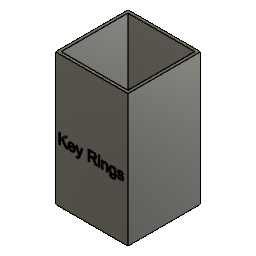
10-32 Box v2 (Autodesk Fusion 360 design; units mm, degrees)
Autodesk Fusion 360 part; units mm, degrees
sketch "Sketch1" plane through (0, 0, 0) normal (0, 1, 0) x (1, 0, 0)
  line L0 (0, 0) -> (50, 0)
  line L1 (50, 0) -> (50, -50)
  line L2 (50, -50) -> (0, -50)
  line L3 (0, -50) -> (0, 0)
  dimension "d1" = 50
  dimension "d2" = 50
  constraint horizontal L0
  constraint vertical L1
  constraint horizontal L2
  constraint vertical L3
  constraint coincident L0.start L3.end
  measures "d1" distance of L0.start L2.end
  measures "d2" distance of L0.start L0.end
extrude "Extrude1" add sketch "Sketch1" along normal blind 1
sketch "Sketch2" plane through (0, 1, 0) normal (0, 1, 0) x (-1, 0, 0)
  line L0 (0, 50) -> (-50, 50)
  line L1 (-50, 50) -> (-50, 0)
  line L2 (-50, 0) -> (0, 0)
  line L3 (0, 0) -> (0, 50)
  line L4 (0, 50) -> (-2, 50)
  line L5 (0, 48) -> (0, 50)
  line L6 (-50, 0) -> (-48, 0)
  line L7 (-50, 2) -> (-50, 0)
  line L8 (-48, 2) -> (-2, 2)
  line L9 (-2, 2) -> (-2, 48)
  line L10 (-2, 48) -> (-48, 48)
  line L11 (-48, 48) -> (-48, 2)
  dimension "d7" = 2
  dimension "d8" = 2
  constraint horizontal L4
  constraint vertical L5
  constraint coincident L0.start L3.end
  constraint horizontal L6
  constraint vertical L7
  constraint coincident L1.end L2.start
  constraint horizontal L8
  constraint vertical L9
  constraint horizontal L10
  constraint vertical L11
  measures "d7" distance of L1.end L7.start
  measures "d8" distance of L1.end L6.end
extrude "Extrude2" add sketch "Sketch2" along normal blind 75
extrude "Extrude3" cut 1 faces at (17.3333, 76, 0.6667) along direction (0, -1, 0) blind 25
sketch "Sketch4" plane through (0, 51, 0) normal (0, 1, 0) x (-1, 0, 0)
  line L0 (-48, 2) -> (-48, 48)
  line L1 (-48, 48) -> (-2, 48)
  line L2 (-2, 48) -> (-2, 2)
  line L3 (-2, 2) -> (-48, 2)
  line L4 (-50, 50) -> (-50, 0)
  line L5 (-50, 0) -> (0, 0)
  line L6 (0, 0) -> (0, 50)
  line L7 (0, 50) -> (-50, 50)
  line L8 (0, 50) -> (2, 50)
  line L9 (2, 50) -> (2, 52)
  line L10 (2, 52) -> (0, 52)
  line L11 (0, 52) -> (0, 50)
  line L12 (-50, 0) -> (-52, 0)
  line L13 (-52, 0) -> (-52, -2)
  line L14 (-52, -2) -> (-50, -2)
  line L15 (-50, -2) -> (-50, 0)
  line L16 (-52, -2) -> (2, -2)
  line L17 (2, -2) -> (2, 52)
  line L18 (2, 52) -> (-52, 52)
  line L19 (-52, 52) -> (-52, -2)
  dimension "d15" = 2
  dimension "d16" = 2
  dimension "d17" = 2
  dimension "d18" = 2
  constraint horizontal L8
  constraint vertical L9
  constraint horizontal L10
  constraint vertical L11
  constraint coincident L6.end L7.start
  constraint horizontal L12
  constraint vertical L13
  constraint horizontal L14
  constraint vertical L15
  constraint coincident L4.end L5.start
  constraint horizontal L16
  constraint vertical L17
  constraint horizontal L18
  constraint vertical L19
  measures "d15" distance of L6.end L8.end
  measures "d16" distance of L6.end L10.end
  measures "d17" distance of L4.end L12.end
  measures "d18" distance of L4.end L14.end
extrude "Extrude15" add 1 faces at (17.3333, 51, 0.6667) along direction (0, 1, 0) blind 40
sketch "Sketch6" plane through (0, 0, 50) normal (0, 0, 1) x (1, 0, 0)
  line L0 (0, 91) -> (0, 0)
  line L1 (0, 0) -> (50, 0)
  line L2 (50, 0) -> (50, 91)
  line L3 (50, 91) -> (0, 91)
  line L4 (2.4671, 35) -> (46.9251, 35) construction
  line L5 (46.9251, 35) -> (46.9251, 45) construction
  line L6 (46.9251, 45) -> (2.4671, 45) construction
  line L7 (2.4671, 45) -> (2.4671, 35) construction
  text T0 "Key Rings" font "Arial" height 10 align ink ink in box 0 x 0 at (2.4771, 35.02) x (1, 0) y (0, 1) spacing 1 height is em
  constraint perpendicular L4 L5
  constraint parallel L4 L6
  constraint parallel L5 L7
extrude "Extrude16" cut sketch "Sketch6" against normal blind 1 text T0
